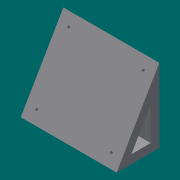
# Autodesk Inventor part: 知能ロボコン土台
Saved by Autodesk Inventor 2013 (Build 170138000, 138)
## iProperties
Created: 2014-08-06
Part Number: 知能ロボコン土台
Material: 一般
Document SubType Name: Modeling
Designer: horumo136
Density: 1 g/cm^3
Author: horumo136
Autodesk Inventor part; units mm, degrees
ref_plane "YZ Plane" through (0, 0, 0) normal (1, 0, 0) x (0, 1, 0)
ref_plane "XZ Plane" through (0, 0, 0) normal (0, 1, 0) x (-1, 0, 0)
ref_plane "XY Plane" through (0, 0, 0) normal (0, 0, 1) x (1, 0, 0)
sketch "スケッチ1" plane through (0, 0, 0) normal (1, 0, 0) x (0, 1, 0)
  line L0 (0, 0) -> (40, 69.282)
  line L1 (0, 0) -> (80, 0) construction
  line L2 (40, 69.282) -> (40, 0)
  line L3 (40, 0) -> (0, 0)
  dimension "d0" = 80
  dimension "d1" = 60
  dimension "d2" = 30
  constraints: 8 end point, 1 equal length, 1 horizontal, 1 perpendicular
  measures "d0" distance of L0.start L0.end
  measures "d1" angle of L1 L0
  measures "d2" angle of L0 L2
extrude "押し出し1" add sketch "スケッチ1" along normal blind 90
sketch "スケッチ2" plane through (0, 0, 0) normal (0, -0.866, 0.5) x (1, 0, 0)
  line L0 (0, 80) -> (10, 80)
  line L1 (10, 80) -> (10, 70)
  line L2 (10, 70) -> (0, 70)
  line L3 (0, 70) -> (0, 80)
  line L4 (90, 80) -> (80, 80)
  line L5 (80, 80) -> (80, 70)
  line L6 (80, 70) -> (90, 70)
  line L7 (90, 70) -> (90, 80)
  line L8 (90, 0) -> (80, 0)
  line L9 (80, 0) -> (80, 10)
  line L10 (80, 10) -> (90, 10)
  line L11 (90, 10) -> (90, 0)
  line L12 (0, 0) -> (10, 0)
  line L13 (10, 0) -> (10, 10)
  line L14 (10, 10) -> (0, 10)
  line L15 (0, 10) -> (0, 0)
  dimension "d5" = 10
  dimension "d6" = 10
  dimension "d7" = 10
  dimension "d8" = 10
  dimension "d9" = 10
  dimension "d10" = 10
  dimension "d11" = 10
  dimension "d12" = 10
  constraints: 32 end point, 8 parallel, 4 coincident, 4 horizontal, 4 perpendicular
  measures "d5" distance of L1.end L2.end
  measures "d6" distance of L0.end L1.end
  measures "d7" distance of L6.end L5.end
  measures "d8" distance of L5.end L4.end
  measures "d9" distance of L9.end L10.end
  measures "d10" distance of L8.end L9.end
  measures "d11" distance of L14.end L13.end
  measures "d12" distance of L13.end L12.end
hole "穴1" at (10, 35, 60.6218) at (10, 5, 8.6603) at (80, 5, 8.6603) at (80, 35, 60.6218) direction (0, 0.866, -0.5) diameter 2.5 depth 20 tip angle 118
sketch "スケッチ3" plane through (0, 0, 0) normal (0, 0, -1) x (-1, 0, 0)
  line L0 (-90, 40) -> (-75, 40)
  line L1 (-75, 40) -> (-75, 30)
  line L2 (-75, 30) -> (-90, 30)
  line L3 (-90, 30) -> (-90, 40)
  line L4 (-90, 0) -> (-75, 0)
  line L5 (-75, 0) -> (-75, 10)
  line L6 (-75, 10) -> (-90, 10)
  line L7 (-90, 10) -> (-90, 0)
  line L8 (0, 40) -> (-15, 40)
  line L9 (-15, 40) -> (-15, 30)
  line L10 (-15, 30) -> (0, 30)
  line L11 (0, 30) -> (0, 40)
  line L12 (0, 0) -> (-15, 0)
  line L13 (-15, 0) -> (-15, 10)
  line L14 (-15, 10) -> (0, 10)
  line L15 (0, 10) -> (0, 0)
  line L16 (-75, 30) -> (-15, 30)
  line L17 (-15, 10) -> (-75, 10)
  point P0 (-45, 10)
  point P1 (-45, 30)
  dimension "d20" = 15
  dimension "d21" = 10
  dimension "d23" = 15
  dimension "d24" = 10
  dimension "d25" = 15
  dimension "d26" = 10
  constraints: 36 end point, 9 parallel, 4 coincident, 4 horizontal, 4 perpendicular, 2 midpoint
  measures "d20" distance of L1.end L2.end
  measures "d21" distance of L0.end L1.end
  measures "d23" distance of L10.end L9.end
  measures "d24" distance of L9.end L8.end
  measures "d25" distance of L13.end L14.end
  measures "d26" distance of L12.end L13.end
hole "穴2" at (75, 30, 0) at (75, 10, 0) at (15, 30, 0) at (15, 10, 0) at (45, 10, 0) at (45, 30, 0) direction (0, 0, 1) diameter 2.5 depth 8 tip angle 118
sketch "スケッチ4" plane through (90, 0, 0) normal (1, 0, 0) x (0, 0, -1)
  line L0 (-69.282, 40) -> (0, 0) projected
  line L1 (0, 0) -> (0, 40) projected
  line L2 (0, 40) -> (-69.282, 40) projected
  line L3 (-8, 40) -> (-8, 4.6188)
  line L4 (0, 32) -> (-55.4256, 32)
  line L5 (-53.282, 40) -> (0, 9.2376)
  point P0 (-39.4256, 32)
  point P1 (-8, 32)
  point P2 (-8, 13.8564)
  dimension "d34" = 8
  dimension "d35" = 8
  dimension "d36" = 8
  constraints: 12 point on line, 6 end point, 1 parallel, 1 perpendicular
  measures "d34" distance between parallel lines of L1 L3
  measures "d35" distance between parallel lines of L4 L2
  measures "d36" distance between parallel lines of L0 L5
extrude "押し出し2" cut sketch "スケッチ4" against normal blind 35 contours L4 L3 L5
sketch "スケッチ5" plane through (0, 0, 0) normal (-1, 0, 0) x (0, 0, 1)
  line L0 (0, 0) -> (69.282, 40) projected
  line L1 (69.282, 40) -> (0, 40) projected
  line L2 (0, 40) -> (0, 0) projected
  line L3 (8, 40) -> (8, 33.1308)
  line L4 (8, 33.1308) -> (8, 4.6188)
  line L5 (0, 32) -> (55.2982, 32)
  line L6 (0, 9.2376) -> (53.282, 40)
  point P0 (39.4256, 32)
  point P1 (8, 32)
  point P2 (8, 13.8564)
  dimension "d39" = 8
  dimension "d40" = 8
  dimension "d41" = 8
  constraints: 11 point on line, 8 end point, 2 perpendicular, 1 collinear, 1 parallel
  measures "d39" distance between parallel lines of L1 L5
  measures "d40" distance between parallel lines of L0 L6
  measures "d41" distance between parallel lines of L2 L4
extrude "押し出し3" cut sketch "スケッチ5" against normal blind 35 contours L4 L5 L6
